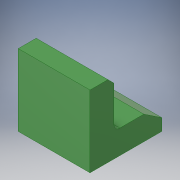
# Autodesk Inventor part: L Chamfer
Saved by Autodesk Inventor 2017 SP1 (Build 210196100, 196)
## iProperties
Created: 2016-12-04
Part Number: L Chamfer
Material: Generic
Document SubType Name: Modeling
Designer: rbibb
Density: 1 g/cm^3
Appearance: Smooth - Dark Forest Green
Author: rbibb
Autodesk Inventor part; units mm, degrees
ref_plane "YZ Plane" through (0, 0, 0) normal (1, 0, 0) x (0, 1, 0)
ref_plane "XZ Plane" through (0, 0, 0) normal (0, 1, 0) x (-1, 0, 0)
ref_plane "XY Plane" through (0, 0, 0) normal (0, 0, 1) x (1, 0, 0)
sketch "Sketch1" plane through (0, 0, 0) normal (1, 0, 0) x (0, 1, 0)
  line L0 (14.2761, 19.3052) -> (-23.8239, 19.3052)
  line L1 (-23.8239, 19.3052) -> (-23.8239, 6.6052)
  line L2 (-23.8239, 6.6052) -> (14.2761, 6.6052)
  line L3 (14.2761, 6.6052) -> (14.2761, 19.3052)
  line L4 (-23.8239, 19.3052) -> (-11.1239, 19.3052)
  line L5 (-11.1239, 19.3052) -> (-11.1239, -18.7948)
  line L6 (-11.1239, -18.7948) -> (-23.8239, -18.7948)
  line L7 (-23.8239, -18.7948) -> (-23.8239, 19.3052)
  point P0 (0, 0)
  dimension "d0" = 38.1
  dimension "d1" = 12.7
  dimension "d2" = 12.7
  dimension "d3" = 38.1
  constraints: 16 end point, 4 parallel, 2 horizontal, 2 perpendicular
  measures "d0" distance of L2.end L1.end
  measures "d1" distance of L1.end L0.end
  measures "d2" distance of L5.end L6.end
  measures "d3" distance of L4.end L5.end
extrude "Extrusion1" add sketch "Sketch1" against normal blind 38.1
chamfer "Chamfer1" distance 3.175 angle 45 1 edges at (-19.05, 14.2761, 6.6052) measured on face at (-12.7, -2.6572, 6.6052)
chamfer "Chamfer2" distance 9.525 distance2 6.35 1 edges at (-19.05, -11.1239, -18.7948) measured on face at (-12.7, -11.1239, -10.3281)
fillet "Fillet1" radius 3.175 1 edges at (-19.05, -11.1239, 6.6052)
body "Solid1"
